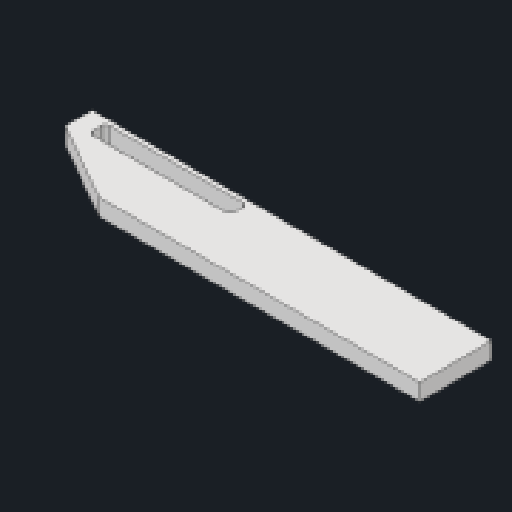
# Autodesk Inventor part: left_hold
Saved by Autodesk Inventor 2023 (Build 270158000, 158)
## iProperties
Created: 2024-04-29
Part Number: left_hold
Material: Generic
Document SubType Name: Modeling
Designer: szymo
Density: 1 g/cm^3
Appearance: Default
Mass: 35.07 g
Surface Area: 127.78 cm^2
Volume: 35.07 cm^3
Author: szymo
Autodesk Inventor part; units mm, degrees
ref_plane "YZ Plane" through (0, 0, 0) normal (1, 0, 0) x (0, 1, 0)
ref_plane "XZ Plane" through (0, 0, 0) normal (0, 1, 0) x (-1, 0, 0)
ref_plane "XY Plane" through (0, 0, 0) normal (0, 0, 1) x (1, 0, 0)
sketch "Sketch1" plane through (0, 0, 0) normal (0, 0, 1) x (1, 0, 0)
  line L0 (91, -34) -> (91, 34) projected
  line L1 (91, 34) -> (41, 34) projected
  line L2 (41, 34) -> (41, 89) projected
  line L3 (41, 89) -> (-91, 89) projected
  line L4 (-91, 89) -> (-91, -89) projected
  line L5 (-91, -89) -> (41, -89) projected
  line L6 (41, -89) -> (41, -34) projected
  line L7 (41, -34) -> (91, -34) projected
  circle A0 centre (-83, 21.5) radius 1.2295 projected
  circle A1 centre (-83, -64.5) radius 1.2295 projected
  circle A2 centre (-83, -21.5) radius 1.2295 projected
  circle A3 centre (-83, 64.5) radius 1.2295 projected
  line L8 (-85, -72) -> (-76, -72) projected
  line L9 (-76, -72) -> (-76, -57) projected
  line L10 (-76, -57) -> (-85, -57) projected
  arc A4 (-87, -55) -> (-85, -57) centre (-85, -55) ccw projected
  line L11 (-87, -55) -> (-87, -31) projected
  arc A5 (-85, -29) -> (-87, -31) centre (-85, -31) ccw projected
  line L12 (-85, -29) -> (-76, -29) projected
  line L13 (-76, -29) -> (-76, -14) projected
  line L14 (-76, -14) -> (-85, -14) projected
  arc A6 (-87, -12) -> (-85, -14) centre (-85, -12) ccw projected
  line L15 (-87, -12) -> (-87, 12) projected
  arc A7 (-85, 14) -> (-87, 12) centre (-85, 12) ccw projected
  line L16 (-85, 14) -> (-76, 14) projected
  line L17 (-76, 14) -> (-76, 29) projected
  line L18 (-76, 29) -> (-85, 29) projected
  arc A8 (-87, 31) -> (-85, 29) centre (-85, 31) ccw projected
  line L19 (-87, 31) -> (-87, 55) projected
  arc A9 (-85, 57) -> (-87, 55) centre (-85, 55) ccw projected
  line L20 (-85, 57) -> (-76, 57) projected
  line L21 (-76, 57) -> (-76, 72) projected
  line L22 (-76, 72) -> (-85, 72) projected
  arc A10 (-87, 74) -> (-85, 72) centre (-85, 74) ccw projected
  line L23 (-87, 74) -> (-87, 89) projected
  line L24 (-91, 89) -> (-87, 89) projected
  line L25 (-91, -89) -> (-91, 89) projected
  line L26 (-91, -89) -> (-87, -89) projected
  line L27 (-87, -89) -> (-87, -74) projected
  arc A11 (-85, -72) -> (-87, -74) centre (-85, -74) ccw projected
  line L28 (60.5, -27) -> (71.5, -27) projected
  line L29 (91, -34) -> (-87, -34)
  line L30 (-87, -34) -> (-87, -27)
  line L31 (-87, -27) -> (91, -27)
  line L32 (91, -27) -> (91, -34)
  line L33 (-91, 89.5) -> (-86.5, 89.5)
  line L34 (-86.5, 89.5) -> (-86.5, 74)
  arc A12 (-86.5, 74) -> (-85, 72.5) centre (-85, 74) ccw
  line L35 (-85, 72.5) -> (-75.5, 72.5)
  line L36 (-75.5, 72.5) -> (-75.5, 56.5)
  line L37 (-75.5, 56.5) -> (-85, 56.5)
  arc A13 (-85, 56.5) -> (-86.5, 55) centre (-85, 55) ccw
  line L38 (-86.5, 55) -> (-86.5, 31)
  arc A14 (-86.5, 31) -> (-85, 29.5) centre (-85, 31) ccw
  line L39 (-85, 29.5) -> (-75.5, 29.5)
  line L40 (-75.5, 29.5) -> (-75.5, 13.5)
  line L41 (-75.5, 13.5) -> (-85, 13.5)
  arc A15 (-85, 13.5) -> (-86.5, 12) centre (-85, 12) ccw
  line L42 (-86.5, 12) -> (-86.5, -12)
  arc A16 (-86.5, -12) -> (-85, -13.5) centre (-85, -12) ccw
  line L43 (-85, -13.5) -> (-75.5, -13.5)
  line L44 (-75.5, -13.5) -> (-75.5, -29.5)
  line L45 (-75.5, -29.5) -> (-85, -29.5)
  arc A17 (-85, -29.5) -> (-86.5, -31) centre (-85, -31) ccw
  line L46 (-86.5, -31) -> (-86.5, -55)
  arc A18 (-86.5, -55) -> (-85, -56.5) centre (-85, -55) ccw
  line L47 (-85, -56.5) -> (-75.5, -56.5)
  line L48 (-75.5, -56.5) -> (-75.5, -72.5)
  line L49 (-75.5, -72.5) -> (-85, -72.5)
  arc A19 (-85, -72.5) -> (-86.5, -74) centre (-85, -74) ccw
  line L50 (-86.5, -74) -> (-86.5, -89.5)
  line L51 (-86.5, -89.5) -> (-91, -89.5)
  line L52 (-87, -31) -> (-75.5, -31)
  line L53 (-75.5, -31) -> (-75.5, -29.5)
  line L54 (-75.5, -31) -> (-75.5, -34)
  point P0 (0, 0)
  point P1 (-76, -27)
  point P2 (-87, -34)
  point P3 (-87, -34)
  point P4 (91, -27)
  point P5 (-75.5, -27)
  dimension "d2" = 0.5
  constraints: 52 end point, 16 point on circle, 8 centre point, 3 perpendicular, 2 collinear, 2 horizontal, 2 parallel, 1 point on line, 26 other
  measures "d2" distance between parallel lines of L12 L45
ref_plane "Work Plane1" through (25, -10, 30) normal (0, 0, 1) x (1, 0, 0)
extrude "Extrusion1" add sketch "Sketch1" along normal up to surface (30 mm away) contours L7 L29 L54 L53 L44 L31 L28 L0
sketch "Sketch2" plane through (-87, -34, 0) normal (0, -1, 0) x (1, 0, 0)
  line L0 (0, 0) -> (0, 4.5) projected
  line L1 (-4, 4.5) -> (0, 4.5) projected
  line L2 (-4, 5.5) -> (-4, 4.5) projected
  line L3 (-18, -3.5) -> (-4, 5.5) projected
  line L4 (-4, -3.5) -> (-18, -3.5) projected
  line L5 (-4, 0) -> (-4, -3.5) projected
  line L6 (0, 0) -> (-4, 0) projected
  line L7 (178, 30) -> (11.5, 30) projected
  line L8 (11.5, 0) -> (178, 0) projected
  line L9 (178, 0) -> (178, 30) projected
  line L10 (0, 4.5) -> (44.1673, 30)
  line L11 (11.5, 0) -> (11.5, 30) projected
  point P0 (87, 0)
  point P1 (11.5, 11.1395)
  dimension "d3" = 30
  constraints: 2 end point, 1 point on line
  measures "d3" angle of L10 L1
extrude "Extrusion3" cut sketch "Sketch2" against normal blind 10 contours L10 L11 L7
sketch "Sketch3" plane through (-75.5, -27, 0) normal (0, 1, 0) x (1, 0, 0)
  arc A0 (66.5, -4) -> (64.5, -2) centre (64.5, -4) ccw projected
  line L0 (9.5, -2) -> (64.5, -2) projected
  arc A1 (9.5, -2) -> (7.5, -4) centre (9.5, -4) ccw projected
  line L1 (7.5, -7.0341) -> (7.5, -4) projected
  arc A2 (7.5, -7.0341) -> (9.5, -9.0341) centre (9.5, -7.0341) ccw projected
  line L2 (64.5, -9.0341) -> (9.5, -9.0341) projected
  arc A3 (64.5, -9.0341) -> (66.5, -7.0341) centre (64.5, -7.0341) ccw projected
  line L3 (66.5, -4) -> (66.5, -7.0341) projected
  constraints: 1 other
extrude "Extrusion4" cut sketch "Sketch3" against normal up to next
body "Solid1"
